Autodesk Fusion 360 part; units mm, degrees
note: some values were not read from the file. Set by a fixed rule: which face or edge a step refers to.
(part 4 of 4)
extrude "Extrude10'" add sketch "Sketch1 (3)" along normal blind 10 from surface at 24 contours A0 | A0 A3 L1 L2 | A4 A5 | A4 A5 | A4 A5 bodies 8 in component "Output"
extrude "Extrude11" cut sketch "Sketch1 (3)" along normal blind 9 from surface at 24 contours A4 A5 | A4 A5 picked at (37.4543, 0.2317) picked at (34.1293, 0.1601) bodies 8 in component "Output"
chamfer "Chamfer3" distance 2 angle 45 1 edges at (33.0972, -0.904, 33) measured on face at (37.9156, -0.2489, 27) on bodies 8 in component "Output"
fillet "Fillet3'" radius 4 2 edges at (14.1421, 5, 29) (14.1421, -5, 29) on bodies 8 in component "Output"
pattern_circular "C-Pattern3" count 6 over 360 about axis through (0, 0, 1.75) along (0, 0, 1) of "Extrude10'", "Extrude11", "Chamfer3", "Fillet3'" in component "Output"
extrude "Extrude5''" add sketch "Sketch1 (3)" along normal blind 15 from surface at 34 contours A3 bodies 8 in component "Output"
extrude "Extrude6''" cut sketch "Sketch1 (3)" against normal blind 1 from surface at 34 contours A4 A5 | A4 A5 picked at (38.4211, 0.2698) picked at (37.4543, 0.2317) bodies 8 in component "Output"
move_face "OffsetFaces1" offset -0.15 6 faces at (-45, -71, 29) (-36.8933, -73.7039, 29) (40, -71, 39) (48.1067, -73.7039, 29) (-48.1067, -73.7039, 39) (36.8933, -73.7039, 39) on bodies 1 in component "Casing"
move_face "OffsetFaces1'" offset -0.15 2 faces at (9.9503, -0.9957, 0.4167) (-9.9503, 0.9957, 40.6667) on bodies 3 4 in component "Shaft"
move_face "OffsetFaces2" offset 0.1 1 faces at (-9.9503, 0.9957, 9.3333) on bodies 3 in component "Shaft"
move_face "OffsetFaces1''" offset -0.25 1 faces at (19.5754, -0.1246, 4) on bodies 7 in component "Output"
move_face "OffsetFaces2'" offset -0.25 1 faces at (-22.1315, 0, 24) on bodies 8 in component "Output"
move_face "OffsetFaces4" offset -0.15 6 faces at (37.9156, -0.2489, 26.5) (18.8545, -32.9062, 28.75) (-19.0704, -32.7816, 28.75) (-37.9156, 0.2489, 26.5) (-18.7422, 32.9603, 26.5) (19.0704, 32.7816, 28.75) on bodies 8 in component "Output"
component "DXF profiles - MEVirtuoso" placed x (1, 0, 0) y (0, 1, 0) z (0, 0, 1) at (0, 0, 0)
component "ACG - Trapezoidal Profiles" placed x (1, 0, 0) y (0, 1, 0) z (0, 0, 1) at (0, 0, 0)
component "Casing" placed x (1, 0, 0) y (0, 1, 0) z (0, 0, 1) at (0, 0, 0)
component "Shaft" placed x (1, 0, 0) y (0, 1, 0) z (0, 0, 1) at (0, 0, 0)
component "Cycloidal Discs" placed x (1, 0, 0) y (0, 1, 0) z (0, 0, 1) at (0, 0, 0)
component "Output" placed x (1, 0, 0) y (0, 1, 0) z (0, 0, 1) at (0, 0, 0)
equation "d63 = 43.20 mm"
equation "d65 = d63"
equation "d66 = eccentricity"
equation "eccentricity = 2.7 mm"
equation "d225 = d227"
equation "d227 = 4 mm"
equation "outer_tooth_height = 4.6 mm"
equation "outer_tooth_end_width = 1.5 mm"
equation "outer_tooth_end_fillet = 1 mm"
equation "outer_tooth_root_fillet = 1 mm"
equation "outer_tooth_root_diam = 110 mm"
equation "outer_tooth_number = 40"
equation "outer_tooth_angle = 25.5 deg"
equation "inner_tooth_end_width = outer_tooth_end_width"
equation "inner_tooth_root_fillet = 1.6 mm"
equation "inner_tooth_root_diam = 95 mm"
equation "inner_tooth_height = 4.6 mm"
equation "inner_tooth_end_fillet = 0.4 mm"
equation "inner_tooth_angle = 20 deg"
equation "inner_tooth_number = 39"
equation "outside_diam = 120 mm"
equation "disc_height = 10 mm"
equation "d261 = 10 mm + 2 * eccentricity"
equation "d262 = d277"
equation "d266 = inner_tooth_end_fillet"
equation "d268 = inner_tooth_root_fillet"
equation "d270 = inner_tooth_number"
equation "d280 = eccentricity"
equation "d282 = outer_tooth_end_fillet"
equation "d284 = outer_tooth_root_fillet"
named bodies: "back", "front", "back (1)"
